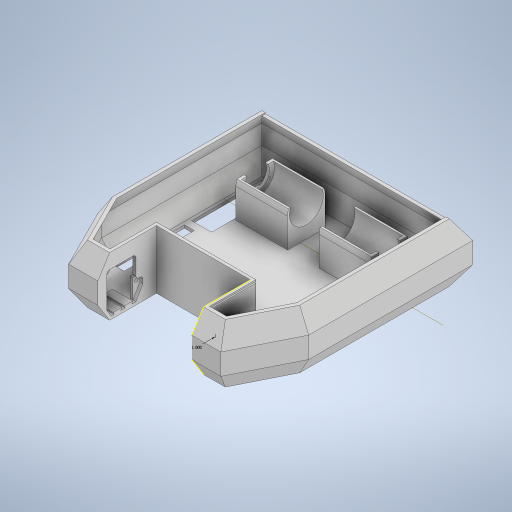
# Autodesk Inventor part: Bot v2 bottom
Saved by Autodesk Inventor 2024 (Build 280153000, 153)
## iProperties
Created: 2023-10-31
Part Number: Bot v2 bottom
Material: Generic
Document SubType Name: Modeling
Designer: CJ110
Density: 1 g/cm^3
Appearance: Default
Author: CJ110
## iProperties of the stored document Bot v2 bottom_3DPrint.ipt
Created: 2023-11-01
Part Number: Bot v2 bottom_3DPrint
Material: Generic
Document SubType Name: Modeling
Designer: CJ110
Density: 1 g/cm^3
Appearance: Default
Author: CJ110
Autodesk Inventor part; units mm, degrees
ref_plane "YZ Plane" through (0, 0, 0) normal (1, 0, 0) x (0, 1, 0)
ref_plane "XZ Plane" through (0, 0, 0) normal (0, 1, 0) x (-1, 0, 0)
ref_plane "XY Plane" through (0, 0, 0) normal (0, 0, 1) x (1, 0, 0)
sketch "Sketch1" plane through (0, 0, 0) normal (0, 1, 0) x (-1, 0, 0)
  line L0 (0, 0) -> (177.8, 0)
  line L1 (177.8, 0) -> (177.8, 228.6)
  line L2 (177.8, 228.6) -> (0, 228.6)
  line L3 (0, 228.6) -> (0, 0)
  line L4 (177.8, 228.6) -> (241.3, 196.85)
  line L5 (241.3, 196.85) -> (241.3, 165.1)
  line L6 (241.3, 165.1) -> (177.8, 165.1)
  line L7 (177.8, 63.5) -> (241.3, 63.5)
  line L8 (241.3, 63.5) -> (241.3, 31.75)
  line L9 (241.3, 31.75) -> (177.8, 0)
  dimension "Bot_Main_Length" = 177.8
  dimension "Bot_Width" = 228.6
  dimension "Weapon_Support_Depth" = 63.5
  dimension "Weapon_Width" = 101.6
  dimension "d4" = 31.75
  dimension "d5" = 31.75
  constraints: 20 end point, 4 point on line, 3 parallel, 2 perpendicular, 1 equal length, 1 horizontal, 1 vertical
  measures "Bot_Main_Length" distance of L2.end L1.end
  measures "Bot_Width" distance of L0.end L1.end
  measures "Weapon_Support_Depth" distance between parallel lines of L1 L5
  measures "Weapon_Width" distance between parallel lines of L7 L6
  measures "d4" distance of L4.end L5.end
  measures "d5" distance of L7.end L8.end
extrude "Extrusion1" add sketch "Sketch1" along normal blind 63.5
chamfer "Chamfer1" distance 12.7 distance2 20.32 7 edges at (-88.9, 63.5, 228.6) (-209.55, 63.5, 212.725) (0, 63.5, 114.3) (-88.9, 63.5, 0) (-209.55, 63.5, 15.875) (-241.3, 63.5, 47.625) (-241.3, 63.5, 180.975) measured on face at (-209.3264, 63.5, 212.2778) measured on face at (-240.8, 63.5, 180.975) measured on face at (-88.9, 63.5, 228.1) measured on face at (-88.9, 63.5, 0.5) measured on face at (-0.5, 63.5, 114.3) measured on face at (-240.8, 63.5, 47.625) measured on face at (-209.3264, 63.5, 16.3222)
chamfer "Chamfer2" distance 12.7 distance2 20.32 7 edges at (-88.9, 0, 228.6) (-209.55, 0, 212.725) (-241.3, 0, 180.975) (-209.55, 0, 15.875) (-241.3, 0, 47.625) (-88.9, 0, 0) (0, 0, 114.3) measured on face at (-240.8, 0, 180.975) measured on face at (-240.8, 0, 47.625) measured on face at (-88.9, 0, 228.1) measured on face at (-88.9, 0, 0.5) measured on face at (-209.3264, 0, 16.3222) measured on face at (-209.3264, 0, 212.2778) measured on face at (-0.5, 0, 114.3)
shell "Shell1" thickness 3.175 removed faces 1 at (-67.7333, 63.5, 97.3667)
sketch "Sketch2" plane through (-174.3865, 3.175, 214.1403) normal (0, 1, 0) x (1, 0, 0)
  line L0 (-3.4135, 3.175) -> (72.7865, 3.175)
  line L1 (72.7865, 3.175) -> (72.7865, 13.97)
  line L2 (72.7865, 13.97) -> (-3.4135, 13.97)
  line L3 (-3.4135, 13.97) -> (-3.4135, 3.175)
  line L4 (80.5518, 3.175) -> (156.7518, 3.175)
  line L5 (156.7518, 3.175) -> (156.7518, 24.765)
  line L6 (156.7518, 24.765) -> (80.5518, 24.765)
  line L7 (80.5518, 24.765) -> (80.5518, 3.175)
  line L8 (159.9268, 0) -> (159.9268, 199.6805) projected
  line L9 (0, 0) -> (159.9268, 0) projected
  line L10 (-0.2385, 45.8653) -> (-0.2385, 153.8153) projected
  line L11 (-0.2385, 99.8403) -> (157.9424, 99.8403) construction
  line L12 (157.9424, 197.6962) -> (157.9424, 1.9844) construction
  line L13 (-52.4537, 45.8653) -> (-52.4537, 26.2269) projected
  line L14 (-52.4537, 26.2269) -> (0, 0) projected
  line L15 (0, 0) -> (159.9268, 0) projected
  line L16 (159.9268, 0) -> (159.9268, 199.6805) projected
  line L17 (159.9268, 199.6805) -> (0, 199.6805) projected
  line L18 (0, 199.6805) -> (-52.4537, 173.4537) projected
  line L19 (-52.4537, 173.4537) -> (-52.4537, 153.8153) projected
  line L20 (-52.4537, 153.8153) -> (-0.2385, 153.8153) projected
  line L21 (-0.2385, 153.8153) -> (-0.2385, 45.8653) projected
  line L22 (-0.2385, 45.8653) -> (-52.4537, 45.8653) projected
  line L23 (-3.4135, 196.5055) -> (72.7865, 196.5055)
  line L24 (72.7865, 196.5055) -> (72.7865, 185.7105)
  line L25 (72.7865, 185.7105) -> (-3.4135, 185.7105)
  line L26 (-3.4135, 185.7105) -> (-3.4135, 196.5055)
  line L27 (80.5518, 196.5055) -> (156.7518, 196.5055)
  line L28 (156.7518, 196.5055) -> (156.7518, 174.9155)
  line L29 (156.7518, 174.9155) -> (80.5518, 174.9155)
  line L30 (80.5518, 174.9155) -> (80.5518, 196.5055)
  point P0 (174.3865, 214.1403)
  dimension "d15" = 21.59
  dimension "d16" = 76.2
  dimension "d17" = 76.2
  dimension "d18" = 3.175
  dimension "d19" = 3.175
  dimension "d20" = 3.175
  dimension "d21" = 10.795
  constraints: 34 end point, 8 symmetric about line, 4 parallel, 2 horizontal, 2 midpoint, 2 perpendicular, 1 collinear
  measures "d15" distance between parallel lines of L6 L4
  measures "d16" distance between parallel lines of L3 L1
  measures "d17" distance between parallel lines of L7 L5
  measures "d18" distance between parallel lines of L8 L5
  measures "d19" distance between parallel lines of L9 L4
  measures "d20" distance between parallel lines of L10 L3
  measures "d21" distance between parallel lines of L0 L2
extrude "Extrusion2" cut sketch "Sketch2" against normal through all contours L3 L2 L1 L0 | L7 L6 L5 L4 | L23 L24 L25 L26 | L27 L28 L29 L30
sketch "Sketch3" plane through (0, 43.18, 228.6) normal (1, 0, 0) x (0, 0, -1)
  line L0 (215.9, 20.32) -> (12.7, 20.32) projected
  line L1 (12.7, 20.32) -> (0, 0) projected
  line L2 (0, 0) -> (228.6, 0) projected
  line L3 (215.9, 20.32) -> (228.6, 0) projected
  line L4 (16.4441, 20.32) -> (14.4597, 17.145)
  line L5 (14.4597, 17.145) -> (214.1403, 17.145)
  line L6 (212.1559, 20.32) -> (214.1403, 17.145)
  point P0 (228.6, -43.18)
  dimension "d24" = 3.175
  dimension "d25" = 3.175
  dimension "d26" = 3.175
  constraints: 6 end point, 2 parallel, 2 point on line, 1 horizontal
  measures "d24" distance between parallel lines of L1 L4
  measures "d25" distance between parallel lines of L0 L5
  measures "d26" distance between parallel lines of L3 L6
extrude "Extrusion3" cut sketch "Sketch3" against normal up to surface contours L6 L5 L4 L0 surface through (-9.0424, 51.6573, 171.45) normal (0.8479983, 0.5299989, 0)
sketch "Sketch4" plane through (-174.625, 3.175, 60.325) normal (1, 0, 0) x (0, 0, -1)
  line L0 (-153.8153, 57.15) -> (-151.8309, 60.325) projected
  line L1 (-151.8309, 60.325) -> (-155.575, 60.325) projected
  line L2 (-155.575, 60.325) -> (-168.275, 40.005) projected
  line L3 (-168.275, 40.005) -> (60.325, 40.005) projected
  line L4 (47.625, 60.325) -> (60.325, 40.005) projected
  line L5 (47.625, 60.325) -> (43.8809, 60.325) projected
  line L6 (43.8809, 60.325) -> (45.8653, 57.15) projected
  line L7 (45.8653, 57.15) -> (-153.8153, 57.15) projected
  line L8 (0, 0) -> (-107.95, 0) projected
  line L9 (0, 0) -> (0, 60.325) projected
  line L10 (-107.95, 60.325) -> (0, 60.325) projected
  line L11 (-107.95, 0) -> (-107.95, 60.325) projected
  line L12 (0, 58.7375) -> (-107.95, 58.7375)
  line L13 (-106.3625, 58.7375) -> (-106.3625, 57.15)
  line L14 (-1.5875, 58.7375) -> (-1.5875, 57.15)
  point P0 (60.325, -3.175)
  point P1 (-107.95, 57.15)
  point P2 (0, 57.15)
  dimension "d29" = 1.5875
  dimension "d30" = 1.5875
  dimension "d31" = 1.5875
  constraints: 6 end point, 6 point on line, 3 perpendicular
  measures "d29" distance between parallel lines of L10 L12
  measures "d30" distance between parallel lines of L11 L13
  measures "d31" distance between parallel lines of L9 L14
extrude "Extrusion4" cut sketch "Sketch4" against normal blind 1.5875 contours L13 L12 L14 L7
extrude "Extrusion5" cut sketch "Sketch4" against normal up to surface contours L11 L12 L13 L7 | L14 L12 L9 L7 surface through (-232.2576, 51.6573, 139.7) normal (-0.8479983, 0.5299989, 0)
sketch "Sketch5" plane through (-174.3865, 3.175, 214.1403) normal (0, 1, 0) x (1, 0, 0)
  line L0 (105.139, 29.845) -> (145.779, 29.845)
  line L1 (145.779, 29.845) -> (145.779, 82.677)
  line L2 (145.779, 82.677) -> (105.139, 82.677)
  line L3 (105.139, 82.677) -> (105.139, 29.845)
  line L4 (118.6518, 259.8603) -> (118.6518, -60.1797) projected
  line L5 (80.5518, 24.765) -> (156.7518, 24.765) projected
  line L6 (-0.2385, 153.8153) -> (-0.2385, 45.8653) projected
  line L7 (-0.2385, 99.8403) -> (159.9268, 99.8403) construction
  line L8 (159.9268, 0) -> (159.9268, 199.6805) projected
  line L9 (105.139, 169.8355) -> (145.779, 169.8355)
  line L10 (145.779, 169.8355) -> (145.779, 117.0035)
  line L11 (145.779, 117.0035) -> (105.139, 117.0035)
  line L12 (105.139, 117.0035) -> (105.139, 169.8355)
  line L13 (125.459, 82.677) -> (125.459, 29.845) construction
  point P0 (174.3865, 214.1403)
  dimension "d36" = 40.64
  dimension "d38" = 52.832
  dimension "d39" = 5.08
  dimension "d40" = 6.8072
  constraints: 20 end point, 4 midpoint, 4 symmetric about line, 2 parallel, 1 horizontal, 1 perpendicular
  measures "d36" distance between parallel lines of L1 L3
  measures "d38" distance between parallel lines of L2 L0
  measures "d39" distance between parallel lines of L5 L0
  measures "d40" distance between parallel lines of L13 L4
extrude "Extrusion6" add sketch "Sketch5" along normal blind 38.1
ref_plane "Work Plane1" through (-177.8, 43.18, 114.3) normal (0, 0, 1) x (1, 0, 0)
sketch "Sketch6" plane through (-177.8, 43.18, 114.3) normal (0, 0, 1) x (1, 0, 0)
  line L0 (149.1925, -40.005) -> (108.5525, -40.005) projected
  line L1 (149.1925, -40.005) -> (149.1925, -1.905) projected
  line L2 (108.5525, -1.905) -> (149.1925, -1.905) projected
  line L3 (108.5525, -40.005) -> (108.5525, -1.905) projected
  arc A0 (111.5869, -1.905) -> (146.158, -1.905) centre (128.8725, -8.255) ccw
  line L4 (149.1925, -1.905) -> (108.5525, -1.905) projected
  line L5 (128.8725, -1.905) -> (128.8725, -40.005) construction
  arc A1 (149.1925, -8.255) -> (148.1748, -1.905) centre (128.8725, -8.255) ccw
  arc A2 (109.5701, -1.905) -> (108.5525, -8.255) centre (128.8725, -8.255) ccw
  point P0 (177.8, -43.18)
  point P1 (111.5869, -1.905)
  point P2 (146.158, -1.905)
  point P3 (148.1748, -1.905)
  point P4 (109.5701, -1.905)
  dimension "d46" = 31.75
  dimension "d47" = 36.83
  constraints: 7 point on line, 6 point on circle, 3 centre point, 2 end point, 2 midpoint, 1 coincident, 1 tangent
  measures "d46" distance from line of L0 A0.centre
  measures "d47" diameter of A0
extrude "Extrusion7" cut sketch "Sketch6" along normal mid plane 142.24 contours A1 L2 L1 | L3 L2 A2 | A0 L2
sketch "Sketch7" plane through (-69.2475, 3.175, 184.2953) normal (0, 0, 1) x (1, 0, 0)
  arc A0 (3.0345, 38.1) -> (37.6055, 38.1) centre (20.32, 31.75) ccw projected
  line L0 (1.0177, 38.1) -> (3.0345, 38.1) projected
  arc A1 (1.0177, 38.1) -> (0, 31.75) centre (20.32, 31.75) ccw projected
  line L1 (0, 0) -> (0, 31.75) projected
  line L2 (40.64, 0) -> (0, 0) projected
  line L3 (40.64, 0) -> (40.64, 31.75) projected
  arc A2 (40.64, 31.75) -> (39.6223, 38.1) centre (20.32, 31.75) ccw projected
  line L4 (37.6055, 38.1) -> (39.6223, 38.1) projected
  circle A3 centre (20.32, 31.75) radius 13.081
  circle A4 centre (20.32, 31.75) radius 18.415
  circle A5 centre (20.32, 16.256) radius 1.143
  line L5 (20.32, 31.75) -> (20.32, 15.113) construction
  line L6 (11.7299, 13.335) -> (28.9101, 13.335) construction
  circle A6 centre (33.7382, 24.003) radius 1.143
  circle A7 centre (33.7382, 39.497) radius 1.143
  circle A8 centre (20.32, 47.244) radius 1.143
  circle A9 centre (6.9018, 39.497) radius 1.143
  circle A10 centre (6.9018, 24.003) radius 1.143
  line L7 (3.0345, 38.1) -> (37.6055, 38.1)
  line L8 (6.9018, 25.6194) -> (7.71, 24.8112)
  line L9 (6.0936, 24.8112) -> (6.9018, 25.6194)
  line L10 (19.5118, 17.0642) -> (20.32, 17.8724)
  line L11 (20.32, 17.8724) -> (21.1282, 17.0642)
  line L12 (32.93, 24.8112) -> (33.7382, 25.6194)
  line L13 (33.7382, 25.6194) -> (34.5464, 24.8112)
  point P0 (69.2475, -3.175)
  point P1 (34.7281, 23.4315)
  point P2 (34.7281, 40.0685)
  point P3 (20.32, 48.387)
  point P4 (5.9119, 40.0685)
  point P5 (5.9119, 23.4315)
  point P6 (31.7563, 38.1)
  point P7 (8.8837, 38.1)
  dimension "d49" = 5.334
  dimension "d50" = 36.83
  dimension "d51" = 2.286
  dimension "d52" = 1.778
  dimension "d55" = 360
  constraints: 18 end point, 9 point on circle, 7 tangent, 5 centre point, 4 vertical alignment, 3 perpendicular, 2 coincident, 1 horizontal, 1 point on line, 1 vertical, 27 other
  measures "d49" radial gap between concentric circles of A4 A3
  measures "d50" diameter of A4
  measures "d51" diameter of A5
  measures "d52" distance from line of L6 L5.end
extrude "Extrusion8" add sketch "Sketch7" along normal blind 3.175 contours L7 A3 A0 | A0 L4 A2 L3 L2 L1 A1 L0
mirror "Mirror1" about plane through (-177.8, 43.18, 114.3) normal (0, 0, 1) of "Extrusion8"
sketch "Sketch12" plane through (-177.8, 0, 63.5) normal (0, 0, 1) x (1, 0, 0)
  line L0 (-53.9115, 47.625) -> (-22.2885, 47.625)
  line L1 (-22.2885, 47.625) -> (-22.2885, 3.175)
  line L2 (-22.2885, 3.175) -> (-49.0403, 3.175)
  line L3 (-53.9115, 10.969) -> (-53.9115, 47.625)
  line L4 (-38.1, 47.625) -> (-38.1, 3.175) construction
  line L5 (-63.5, 20.32) -> (-63.5, 43.18) projected
  line L6 (-49.0403, 3.175) -> (3.4135, 3.175) projected
  line L7 (3.4135, 3.175) -> (163.3403, 3.175) projected
  line L8 (163.3403, 3.175) -> (3.4135, 3.175) projected
  line L9 (3.4135, 3.175) -> (-49.0403, 3.175) projected
  line L10 (-49.0403, 3.175) -> (3.175, 3.175) projected
  line L11 (3.175, 3.175) -> (-49.0403, 3.175) projected
  line L12 (0, 3.175) -> (76.2, 3.175) projected
  line L13 (76.2, 3.175) -> (0, 3.175) projected
  line L14 (83.9653, 3.175) -> (160.1653, 3.175) projected
  line L15 (160.1653, 3.175) -> (83.9653, 3.175) projected
  line L16 (83.9653, 3.175) -> (160.1653, 3.175) projected
  line L17 (160.1653, 3.175) -> (83.9653, 3.175) projected
  line L18 (0, 3.175) -> (76.2, 3.175) projected
  line L19 (76.2, 3.175) -> (0, 3.175) projected
  line L20 (108.5525, 3.175) -> (149.1925, 3.175) projected
  line L21 (149.1925, 3.175) -> (108.5525, 3.175) projected
  line L22 (108.5525, 3.175) -> (149.1925, 3.175) projected
  line L23 (149.1925, 3.175) -> (108.5525, 3.175) projected
  line L24 (-49.0403, 3.175) -> (-60.325, 21.2306) projected
  line L25 (-49.0403, 3.175) -> (-60.325, 21.2306) projected
  point P0 (177.8, 0)
  point P1 (-38.1, 31.75)
  point P2 (-38.1, 31.75)
  point P3 (-53.9115, 10.969)
  dimension "d80" = 31.623
  dimension "d81" = 25.4
  dimension "d83" = 44.45
  constraints: 10 end point, 3 point on line, 2 parallel, 1 coincident, 1 collinear, 1 horizontal, 1 midpoint, 1 perpendicular
  measures "d80" distance between parallel lines of L1 L3
  measures "d81" distance between parallel lines of L5 L4
  measures "d83" distance between parallel lines of L2 L0
extrude "Extrusion12" cut sketch "Sketch12" against normal up to next
fillet "Fillet1" radius 3.175 2 edges at (-231.7115, 47.625, 61.9125) (-200.0885, 47.625, 61.9125)
sketch "Sketch13" plane through (-177.8, 0, 63.5) normal (0, 0, 1) x (1, 0, 0)
  line L0 (-38.1, 47.625) -> (-38.1, 3.175) construction
  line L1 (-49.0403, 3.175) -> (-53.9115, 10.969) projected
  line L2 (-53.9115, 10.969) -> (-53.9115, 44.45) projected
  line L3 (-22.2885, 44.45) -> (-22.2885, 3.175) projected
  line L4 (-22.2885, 3.175) -> (-49.0403, 3.175) projected
  line L5 (-50.8, 0) -> (-63.5, 20.32) projected
  line L6 (-50.8, 0) -> (0, 0) projected
  line L7 (0, 0) -> (0, 63.5) projected
  line L8 (-50.8, 63.5) -> (0, 63.5) projected
  line L9 (-63.5, 43.18) -> (-50.8, 63.5) projected
  line L10 (-63.5, 20.32) -> (-63.5, 43.18) projected
  line L11 (-22.2885, 3.175) -> (-49.0403, 3.175) projected
  line L12 (-34.0843, 3.175) -> (-35.0368, 5.715)
  line L13 (-35.0368, 5.715) -> (-25.5118, 5.715)
  line L14 (-25.5118, 5.715) -> (-26.4643, 3.175)
  line L15 (-46.1493, 3.175) -> (-47.1018, 5.715)
  line L16 (-47.1018, 5.715) -> (-37.5768, 5.715)
  line L17 (-37.5768, 5.715) -> (-38.5293, 3.175)
  line L18 (-38.6649, 3.175) -> (-37.76, 5.588)
  line L19 (-37.76, 5.588) -> (-46.9185, 5.588)
  line L20 (-46.9185, 5.588) -> (-46.0136, 3.175)
  line L21 (-26.5999, 3.175) -> (-25.695, 5.588)
  line L22 (-25.695, 5.588) -> (-34.8535, 5.588)
  line L23 (-34.8535, 5.588) -> (-33.9486, 3.175)
  line L24 (-50.7365, 47.625) -> (-25.4635, 47.625) projected
  arc A0 (-22.2885, 44.45) -> (-25.4635, 47.625) centre (-25.4635, 44.45) ccw projected
  arc A1 (-50.7365, 47.625) -> (-53.9115, 44.45) centre (-50.7365, 44.45) ccw projected
  point P0 (177.8, 0)
  point P1 (-30.2743, 5.715)
  dimension "d87" = 7.8257
  dimension "d88" = 7.62
  dimension "d89" = 2.54
  dimension "d90" = 9.525
  dimension "d91" = 2.54
  dimension "d92" = 2.54
  dimension "d93" = 0.127
  dimension "d94" = 0.127
  dimension "d95" = 0.127
  dimension "d96" = 0.127
  dimension "d97" = 0.127
  dimension "d98" = 0.127
  constraints: 26 end point, 4 equal length, 2 horizontal, 1 collinear, 1 midpoint, 1 point on line, 1 vertical, 9 other
  measures "d87" distance from line of L0 point (-30.274, 5.715)
  measures "d88" distance of L14.end L12.start
  measures "d90" distance of L13.end L12.end
  measures "d91" distance between parallel lines of L4 L16
  measures "d92" distance of L12.end L16.end
  measures "d93" distance between parallel lines of L16 L19
  measures "d94" distance between parallel lines of L13 L22
  measures "d95" distance between parallel lines of L12 L23
  measures "d96" distance between parallel lines of L14 L21
  measures "d97" distance between parallel lines of L17 L18
  measures "d98" distance between parallel lines of L15 L20
extrude "Extrusion13" add sketch "Sketch13" against normal blind 22 contours L20 L19 L18 L4 | L23 L22 L21 L4
sketch "Sketch15" plane through (-238.125, 21.2306, 60.325) normal (0, 0, -1) x (-1, 0, 0)
  line L0 (-6.4135, 23.2194) -> (-6.4135, -10.2616) projected
  line L1 (-6.4135, -10.2616) -> (0, 0) projected
  line L2 (0, 0) -> (0, 21.0388) projected
  line L3 (0, 21.0388) -> (-11.2847, 39.0944) projected
  line L4 (-11.2847, 39.0944) -> (-63.5, 39.0944) projected
  line L5 (-63.5, -18.0556) -> (-63.5, 39.0944) projected
  line L6 (-38.0365, -18.0556) -> (-63.5, -18.0556) projected
  line L7 (-38.0365, -18.0556) -> (-38.0365, 23.2194) projected
  arc A0 (-34.8615, 26.3944) -> (-38.0365, 23.2194) centre (-34.8615, 23.2194) ccw projected
  line L8 (-34.8615, 26.3944) -> (-9.5885, 26.3944) projected
  arc A1 (-6.4135, 23.2194) -> (-9.5885, 26.3944) centre (-9.5885, 23.2194) ccw projected
  line L9 (-38.0365, -18.0556) -> (-45.6565, -4.8574)
  line L10 (-45.6565, -4.8574) -> (-45.6565, 2.7626)
  line L11 (-45.6565, 2.7626) -> (-38.0365, 2.7626)
  circle A2 centre (-41.8084, -1.0474) radius 1.5875
  line L12 (-45.6565, -4.8574) -> (-45.6565, -18.0556)
  point P0 (-238.125, -21.2306)
  point P1 (-22.225, 26.3944)
  dimension "d107" = 7.62
  dimension "d108" = 7.62
  dimension "d109" = 30
  dimension "d110" = 3.175
  dimension "d112" = 3.81
  dimension "d122" = 19.5834
  constraints: 8 end point, 2 perpendicular, 2 point on line, 1 centre point, 1 midpoint, 1 vertical
  measures "d107" distance of L10.end L11.end
  measures "d108" distance of L9.end L10.end
  measures "d109" angle of L7 L9
  measures "d110" diameter of A2
  measures "d112" distance from line of L11 A2.centre
  measures "d122" horizontal distance of A2.centre point (-22.225, 26.394)
extrude "Extrusion14" cut sketch "Sketch15" against normal up to surface (3.175 mm away) contours L7 L9 L10 L11 | A2
fillet "Fillet2" radius 3.175 2 edges at (-192.4685, 23.9932, 61.9125) (-200.0885, 23.9932, 61.9125)
extrude "Extrusion15" add sketch "Sketch15" along normal blind 3.175 contours L7 L9 L10 L11 | L6 L12 L9 | A2
fillet "Fillet3" radius 3.175 1 edges at (-192.4685, 3.175, 58.7375)
sketch "Sketch16" plane through (-177.8, 0, 165.1) normal (0, 0, -1) x (-1, 0, 0)
  circle A0 centre (38.1, 31.75) radius 4.7323
  line L0 (63.5, 20.32) -> (63.5, 43.18) projected
  line L1 (63.5, 31.75) -> (0, 31.75) construction
  line L2 (0, 0) -> (0, 63.5) projected
  line L3 (63.5, 20.32) -> (50.8, 0) projected
  line L4 (63.5, 20.32) -> (63.5, 43.18) projected
  line L5 (50.8, 63.5) -> (63.5, 43.18) projected
  line L6 (0, 63.5) -> (50.8, 63.5) projected
  line L7 (0, 0) -> (0, 63.5) projected
  line L8 (0, 0) -> (50.8, 0) projected
  point P0 (-177.8, 0)
  dimension "d123" = 25.4
  constraints: 2 end point, 2 midpoint, 1 centre point, 1 point on line
  measures "d123" distance from line of L0 A0.centre
hole "Hole1" at (-196.3166, 20.1832, 60.325) direction (0, 0, -1) diameter 4 depth 3.175 clearance for "Hex Head Machine Screw" size "M4" standard "Ansi Metric M Profile"
sketch "Sketch8" plane through (-177.8, 0, 63.5) normal (0, 0, 1) x (1, 0, 0)
  line L0 (-63.5, 20.32) -> (-63.5, 43.18) projected
  line L1 (-63.5, 31.75) -> (-0.3806, 31.75) construction
  line L2 (-50.8, 63.5) -> (2.9981, 63.5) projected
  line L3 (-38.1, 63.5) -> (-38.1, 0) construction
  line L4 (-50.8, 0) -> (0, 0) projected
  line L5 (-50.8, 0) -> (-63.5, 20.32) projected
  line L6 (-50.8, 0) -> (0, 0) projected
  line L7 (0, 0) -> (0, 63.5) projected
  line L8 (-50.8, 63.5) -> (0, 63.5) projected
  line L9 (-63.5, 43.18) -> (-50.8, 63.5) projected
  line L10 (-63.5, 20.32) -> (-63.5, 43.18) projected
  circle A0 centre (-38.1, 31.75) radius 13.127
  arc A1 (-46.8557, 46.0735) -> (-52.4235, 40.5057) centre (-49.6396, 43.2896) ccw
  line L11 (-52.4235, 40.5057) -> (-49.7388, 37.821)
  line L12 (-46.8557, 46.0735) -> (-44.171, 43.3888)
  line L13 (-38.1, 31.75) -> (-52.4235, 46.0735) construction
  line L14 (-52.4235, 22.9943) -> (-49.7388, 25.679)
  line L15 (-38.1, 31.75) -> (-52.4235, 17.4265) construction
  arc A2 (-52.4235, 22.9943) -> (-46.8557, 17.4265) centre (-49.6396, 20.2104) ccw
  line L16 (-46.8557, 17.4265) -> (-44.171, 20.1112)
  line L17 (-29.3443, 17.4265) -> (-32.029, 20.1112)
  line L18 (-38.1, 31.75) -> (-23.7765, 17.4265) construction
  arc A3 (-29.3443, 17.4265) -> (-23.7765, 22.9943) centre (-26.5604, 20.2104) ccw
  line L19 (-23.7765, 22.9943) -> (-26.4612, 25.679)
  line L20 (-23.7765, 40.5057) -> (-26.4612, 37.821)
  line L21 (-38.1, 31.75) -> (-23.7765, 46.0735) construction
  arc A4 (-23.7765, 40.5057) -> (-29.3443, 46.0735) centre (-26.5604, 43.2896) ccw
  line L22 (-29.3443, 46.0735) -> (-32.029, 43.3888)
  point P0 (177.8, 0)
  point P1 (-49.7388, 25.679)
  point P2 (-44.171, 20.1112)
  point P3 (-32.029, 20.1112)
  point P4 (-26.4612, 25.679)
  point P5 (-26.4612, 37.821)
  dimension "d60" = 25.4
  dimension "d61" = 26.254
  dimension "d62" = 7.874
  dimension "d63" = 45
  dimension "d64" = 16.3195
  dimension "d67" = 360
  constraints: 28 end point, 11 point on circle, 5 centre point, 2 coincident, 2 midpoint, 2 parallel, 2 point on line, 2 tangent, 1 horizontal, 1 vertical, 43 other
  measures "d60" distance between parallel lines of L3 L0
  measures "d61" diameter of A0
  measures "d62" diameter of A1
  measures "d63" angle of L1 L13
  measures "d64" distance of L13.start A1.centre
equation "\"d18\" = Wall_Thickness"
equation "\"d19\" = d18"
equation "\"d20\" = Wall_Thickness"
equation "\"d21\" = 0.5 * d15"
equation "\"d24\" = Wall_Thickness"
equation "\"d25\" = Wall_Thickness"
equation "\"d26\" = Wall_Thickness"
equation "\"d29\" = 0.5 * Wall_Thickness"
equation "\"d30\" = 0.5 * Wall_Thickness"
equation "\"d31\" = 0.5 * Wall_Thickness"
equation "\"d46\" = 0.5 * Wall_Height"
equation "\"Wall_Thickness\" = 3.175"
equation "\"Wall_Height\" = 63.5"
equation "\"Wheel_Hole_Diameter\" = 79.375"
equation "\"Driven_Wheel_Width\" = 23.495"
equation "\"Brushless_Diameter\" = 26"
body "Solid1"
